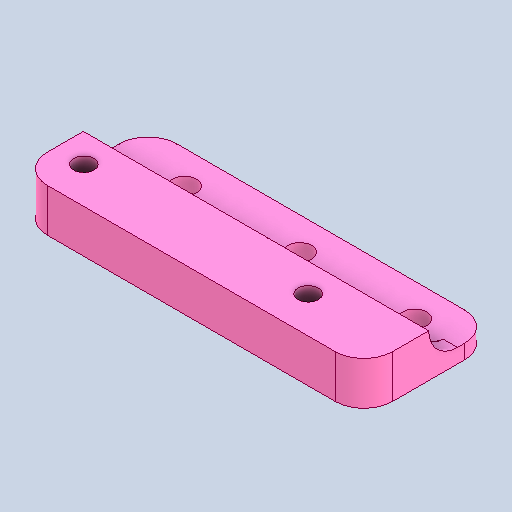
# Autodesk Inventor part: DriveMotorMount5
Saved by Autodesk Inventor 2025.1 (Build 291241020, 241B)
## iProperties
Created: 2023-04-07
Part Number: DriveMotorMount5
Material: Generic
Document SubType Name: Modeling
Designer: Dave
Density: 1 g/cm^3
Appearance: Pink
Author: Dave
Autodesk Inventor part; units mm, degrees
ref_plane "YZ Plane" through (0, 0, 0) normal (1, 0, 0) x (0, 1, 0)
ref_plane "XZ Plane" through (0, 0, 0) normal (0, 1, 0) x (-1, 0, 0)
ref_plane "XY Plane" through (0, 0, 0) normal (0, 0, 1) x (1, 0, 0)
sketch "Sketch1" plane through (0, 0, 0) normal (1, 0, 0) x (0, 1, 0)
  line L0 (0, 0) -> (0, -28.575)
  line L1 (0, -28.575) -> (3.175, -28.575)
  line L2 (3.175, -28.575) -> (3.175, -14.2875)
  line L3 (3.175, -14.2875) -> (9.525, -14.2875)
  line L4 (9.525, -14.2875) -> (9.525, 0)
  line L5 (9.525, 0) -> (0, 0)
  point P0 (0, -14.2875)
  dimension "d0" = 3.175
  dimension "d1" = 9.525
  dimension "d2" = 28.575
  constraints: 12 end point, 5 perpendicular, 1 horizontal alignment, 1 midpoint, 1 vertical
  measures "d0" distance of L0.end L1.end
  measures "d1" distance of L4.end L0.start
  measures "d2" distance of L0.start L0.end
extrude "Extrusion1" add sketch "Sketch1" along normal blind 76.2
sketch "Sketch2" plane through (0, 9.525, 0) normal (0, 1, 0) x (1, 0, 0)
  circle A0 centre (15.2237, 21.3995) radius 2.65
  circle A1 centre (40.6237, 21.3995) radius 2.65
  circle A2 centre (66.0237, 21.3995) radius 2.65
  circle A3 centre (55.8475, 8.0485) radius 2.25
  circle A4 centre (6.35, 8.0485) radius 2.25
  line L0 (0, 28.575) -> (0, 14.2875) projected
  line L1 (0, 14.2875) -> (0, 0) projected
  line L2 (0, 14.2875) -> (76.2, 14.2875) projected
  point P0 (0, 21.4313)
  point P1 (0, 7.1438)
  dimension "d5" = 5.3
  dimension "d6" = 25.4
  dimension "d7" = 25.4
  dimension "d8" = 49.4975
  dimension "d9" = 4.5
  dimension "d10" = 13.351
  dimension "d11" = 8.8737
  dimension "d13" = 7.112
  dimension "d14" = 6.35
  constraints: 5 centre point, 3 equal radius, 3 horizontal alignment, 2 midpoint
  measures "d5" diameter of A0
  measures "d6" distance of A0.centre A1.centre
  measures "d7" distance of A1.centre A2.centre
  measures "d8" distance of A3.centre A4.centre
  measures "d9" diameter of A4
  measures "d10" vertical distance of A4.centre A0.centre
  measures "d11" horizontal distance of A0.centre A4.centre
  measures "d13" distance from line of L2 A0.centre
  measures "d14" distance from line of L1 A4.centre
extrude "Extrusion2" cut sketch "Sketch2" against normal through all
sketch "Sketch3" plane through (0, 0, -28.575) normal (0, -1, 0) x (1, 0, 0)
  circle A0 centre (55.8475, 20.5265) radius 2.25 projected
  circle A1 centre (55.8475, 20.5265) radius 2.625
  circle A2 centre (6.35, 20.5265) radius 2.25 projected
  circle A3 centre (6.35, 20.5265) radius 2.625
  point P0 (0, 28.575)
  dimension "d17" = 5.25
  dimension "d18" = 5.25
  constraints: 2 centre point, 2 coincident
  measures "d17" diameter of A1
  measures "d18" diameter of A3
extrude "Extrusion3" cut sketch "Sketch3" against normal blind 5
fillet "Fillet1" radius 6.35 5 edges at (76.2, 4.7625, 0) (38.1, 3.175, -14.2875) (76.2, 1.5875, -28.575) (0, 1.5875, -28.575) (0, 4.7625, 0)
sketch "Sketch4" plane through (0, 9.525, -6.35) normal (0, 1, 0) x (1, 0, 0)
  arc A0 (6.35, 22.225) -> (0, 15.875) centre (6.35, 15.875) ccw projected
  line L0 (0, 15.875) -> (0, 14.2875) projected
  line L1 (12.6857, 14.2875) -> (0, 14.2875) projected
  arc A1 (17.7618, 14.2875) -> (12.6857, 14.2875) centre (15.2237, 15.0495) ccw projected
  line L2 (38.0857, 14.2875) -> (17.7618, 14.2875) projected
  arc A2 (43.1618, 14.2875) -> (38.0857, 14.2875) centre (40.6237, 15.0495) ccw projected
  line L3 (63.4857, 14.2875) -> (43.1618, 14.2875) projected
  arc A3 (68.5618, 14.2875) -> (63.4857, 14.2875) centre (66.0237, 15.0495) ccw projected
  line L4 (76.2, 14.2875) -> (68.5618, 14.2875) projected
  line L5 (76.2, 15.875) -> (76.2, 14.2875) projected
  arc A4 (76.2, 15.875) -> (69.85, 22.225) centre (69.85, 15.875) ccw projected
  line L6 (6.35, 22.225) -> (69.85, 22.225) projected
  circle A5 centre (15.2237, 15.0495) radius 7.112
  circle A6 centre (40.6237, 15.0495) radius 7.112
  circle A7 centre (66.0237, 15.0495) radius 7.112
  point P0 (0, -6.35)
  dimension "d22" = 14.224
  dimension "d23" = 14.224
  dimension "d24" = 14.224
  constraints: 3 centre point, 3 coincident
  measures "d22" diameter of A5
  measures "d23" diameter of A6
  measures "d24" diameter of A7
extrude "Extrusion4" cut sketch "Sketch4" against normal up to surface (6.35 mm away) contours A5 L2 A1 L1 | L1 A1 L2 A5 | A7 L3 A3 L4 | L4 A3 L3 A7 | A6 L3 A2 L2 | L2 A2 L3 A6
equation "\"d7\" = d6"
body "Solid1"
